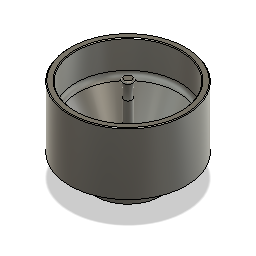
P100_Hot_Load_Funnel (Autodesk Fusion 360 design; units mm, degrees)
Autodesk Fusion 360 part; units mm, degrees
sketch "Sketch1" plane through (0, 0, 0) normal (0, 0, 1) x (1, 0, 0)
  line L0 (0, 0) -> (-35, 0)
  line L1 (-35, 0) -> (-35, 2.5)
  line L2 (-35, 2.5) -> (-39, 2.5)
  line L3 (-39, 2.5) -> (-39, 7.5)
  line L4 (-39, 7.5) -> (-39, 12.5)
  line L5 (-39, 12.5) -> (0, 12.5)
  line L6 (0, 12.5) -> (0, 0)
  line L7 (-39, 12.5) -> (-35, 12.5)
  line L8 (-35, 12.5) -> (-27.7831, 0)
  line L9 (-35.5774, 12.5) -> (-28.3605, 0)
  line L10 (-35, 0) -> (-34, 0) construction
  line L11 (-35, 12.5) -> (-19.3037, -14.6868)
  line L12 (-35.5774, 12.5) -> (-19.8811, -14.6868)
  line L13 (-19.3037, -14.6868) -> (-19.8811, -14.6868)
  line L14 (0, 12.5) -> (-4, 12.5)
  circle A0 centre (-18.149, -12.6868) radius 2
  arc A1 (-18.8484, -10.8131) -> (-4, 20.5) centre (-27.5463, 12.4884) ccw
  line L15 (-19.3037, -14.6868) -> (0, -14.6868)
  line L16 (0, -14.6868) -> (0, 0)
  line L17 (-4, 12.5) -> (-4, 20.5)
  line L18 (0, 12.5) -> (0, 20.5)
  line L19 (0, 20.5) -> (-4, 20.5)
  line L20 (0, 16.5) -> (-3, 16.5)
  line L21 (-39, 12.5) -> (-39, 25.5)
  line L22 (-39, 25.5) -> (0, 25.5)
  line L23 (0, 25.5) -> (0, 20.5)
  line L24 (-4, 20.5) -> (-33, 20.5)
  line L25 (-35, 0) -> (-28.8618, -14.6868)
  line L26 (-28.8618, -14.6868) -> (-19.8811, -14.6868)
  line L27 (-35, 12.5) -> (-35, 19)
  line L28 (-35, 19) -> (-39, 19)
  line L29 (-33, 20.5) -> (-33, 12.5)
  line L30 (-35, 19) -> (0, 19)
  line L31 (-35, 19) -> (-34.8, 19)
  line L32 (-34.8, 19) -> (-34.8, 12.5)
  line L33 (-19.8811, -13.6868) -> (-19.8811, -14.6868)
  line L34 (-18.149, -12.6868) -> (-20.4584, -12.6868)
  line L35 (-28.8618, -14.6868) -> (-28.8618, -26.1449)
  arc A2 (-18.56, -18.617) -> (-19.8811, -13.6868) centre (-28.4205, -18.617) ccw
  line L36 (-18.56, -18.617) -> (-18.56, -22.5613)
  line L37 (-18.56, -22.5613) -> (-28.8618, -22.5613)
  line L38 (-28.8618, -22.5613) -> (-28.8618, -26.1449)
  line L39 (-18.56, -22.5613) -> (0, -22.5613)
  line L40 (0, -22.5613) -> (0, -14.6868)
  line L41 (-19.3771, -14.6868) -> (-28.8618, -14.6868)
  line L42 (-18.56, -22.5613) -> (-21.5, -22.5613)
  line L43 (-21.5, -22.5613) -> (-21.5, -22.1613)
  arc A3 (-21.5, -22.1613) -> (-28.8618, -14.6868) centre (-28.9754, -22.1613) ccw
  circle A4 centre (-18.149, -12.6868) radius 1.8
  line L44 (-20.0811, -12.9897) -> (-20.0811, -14.6868)
  arc A5 (-18.36, -18.617) -> (-20.0811, -12.9897) centre (-28.4205, -18.617) ccw
  line L45 (-18.36, -18.617) -> (-18.36, -22.5613)
  arc A6 (-18.7785, -11.0004) -> (-3.8107, 20.5644) centre (-27.5463, 12.4884) ccw
  line L46 (-39, 7.5) -> (-35, 7.5)
  line L47 (-35, 7.5) -> (-35, 2.5)
  line L48 (-35, 5) -> (-39, 5)
  line L49 (-28.8618, -14.6868) -> (-39, -7.5351)
  line L50 (-35, 0) -> (-35, -10.3567)
  line L51 (-39, 2.5) -> (-39, -7.5351)
  line L52 (-28.8618, -14.6868) -> (-17.6989, -22.5613)
  line L53 (-21.5, -22.5613) -> (-21.5, -19.8799)
  dimension "d1" = 35
  dimension "d4" = 2.5
  dimension "d5" = 4
  dimension "d6" = 5
  dimension "d7" = 5
  dimension "d8" = 4
  dimension "d9" = 120
  dimension "d10" = 0.5
  dimension "d17" = 4
  dimension "d20" = 8
  dimension "d21" = 4
  dimension "d22" = 3
  dimension "d23" = 13
  dimension "d42" = 6.5
  dimension "d43" = 2
  dimension "d44" = 0.2
  dimension "d147" = 4
  dimension "d148" = 2.94
  dimension "d150" = 0.4
  dimension "d151" = -0.2
  dimension "d152" = 0.2
  dimension "d153" = 0.2
  dimension "d168" = 35.2
  dimension "d176" = 21.5
  constraint coincident L0.start L6.end
  constraint horizontal L0
  constraint perpendicular L0 L1
  constraint perpendicular L1 L2
  constraint perpendicular L2 L3
  constraint parallel L3 L4
  constraint perpendicular L4 L5
  constraint perpendicular L5 L6
  constraint perpendicular L4 L7
  constraint coincident L0 L8.end
  constraint coincident L7 L9.start
  constraint coincident L0 L9.end
  constraint parallel L8 L9
  constraint horizontal L10
  constraint parallel L8 L11
  constraint parallel L9 L12
  constraint coincident L12 L13.end
  constraint horizontal L13
  constraint coincident L12.end L13.end
  constraint perpendicular L6 L14
  constraint tangent L11 A0
  constraint perpendicular L0 L16
  constraint perpendicular L14 L17
  constraint perpendicular L14 L18
  constraint coincident L18 L19.start
  constraint horizontal L19
  constraint midpoint L18 L20.start
  constraint coincident A1 L20.end
  constraint perpendicular L18 L20
  constraint perpendicular L7 L21
  constraint perpendicular L21 L22
  constraint perpendicular L19 L23
  constraint perpendicular L17 L24
  constraint parallel L13 L26
  constraint coincident A0 A1.start
  constraint tangent A0 A1
  constraint horizontal L15
  constraint perpendicular L7 L27
  constraint midpoint L21 L28.end
  constraint coincident L5 L29.end
  constraint perpendicular L5 L29
  constraint perpendicular L27 L30
  constraint coincident L18 L30.end
  constraint perpendicular L27 L31
  constraint perpendicular L30 L32
  constraint coincident A0 L33.start
  constraint coincident L26 L12.end
  constraint perpendicular L26 L33
  constraint coincident A0.centre L34.start
  constraint coincident L11 L34.end
  constraint horizontal L34
  constraint tangent A0 L15
  constraint perpendicular L26 L35
  constraint tangent L11 A2
  constraint vertical L36
  constraint tangent A2 L36
  constraint perpendicular L36 L37
  constraint vertical L38
  constraint perpendicular L36 L39
  constraint perpendicular L15 L40
  constraint coincident A2 L41.start
  constraint coincident L13 L41.start
  constraint perpendicular L36 L42
  constraint perpendicular L42 L43
  constraint tangent L43 A3
  constraint perpendicular L4 L46
  constraint midpoint L47 L48.start
  constraint midpoint L3 L48.end
  constraint coincident L49 L50.end
  constraint perpendicular L0 L50
  constraint coincident L1 L0.end
  constraint coincident L49 L51.end
  constraint perpendicular L2 L51
  constraint coincident L39 L52.end
  constraint parallel L49 L52
  constraint coincident L52 L53.end
  constraint perpendicular L42 L53
  measures "d1" distance of L0.start L0.end
  measures "d4" distance of L0.end L1.end
  measures "d5" distance of L1.end L2.end
  measures "d6" distance of L2.end L3.end
  measures "d7" distance of L3.end L4.end
  measures "d8" distance of L4.end L7.end
  measures "d9" angle of L5 L8
  measures "d10" distance of L8 L9
  measures "d17" diameter of A0
  measures "d20" distance of L14.end A1.end
  measures "d21" distance of A1.end L18.end
  measures "d22" distance of L20.start L20.end
  measures "d23" distance of L4.end L21.end
  measures "d42" distance of L7.end L27.end
  measures "d43" distance of L27 L29
  measures "d44" distance of L27.end L31.end
  measures "d147" distance of L11.end A2.start
  measures "d148" distance of L36.end L42.end
  measures "d150" distance of L42.end L43.end
  measures "d168" angle of L15 L49
  measures "d176" distance of L39.end L42.end
revolve "Revolve1" add sketch "Sketch1" angle 360 about axis through (0, 12.5, 0) along (0, -1, 0) contours L0 L11 L12 L44 | L0 L5 L7 L8 L9 L11 L12 | L0 L12 L25 L26 L41 L44 | L0 L1 L4 L5 L7 L9 L12 L46 L47 | L5 L7 L21 L27 L28 | L1 L2 L49 L50 L51 | L25 L49 L50 | L11 L12 L33 L44 | L12 L26 L41 L44 | L2 L3 L47 L48 | L13 L26 A2 L36 L41 A3 L52 | A3 L52 | L13 L33 A2 L41 | L3 L46 L47 L48 | L36 L37 L42 L43 L52 L53 makes body 1
revolve "Revolve2" add sketch "Sketch1" angle 360 about axis through (0, -14.6868, 0) along (0, 1, 0) separate body contours L0 L5 L6 L14 A6 | L0 A0 L15 L16 A6 | A0 A4 A5 A6 | L5 L14 L18 L20 A6 | A4 | L15 L39 L40 A5 L45 L52 | L18 L20 L30 A6 | A0 L15 A5 | L18 L19 L30 A6 | L39 L45 L52 makes body 2
revolve "Revolve3" add sketch "Sketch1" angle 360 about axis through (0, 12.5, 0) along (0, 1, 0) separate body contours L19 L21 L22 L23 L24 L28 L29 L30 L31 | L17 L24 L29 L30 makes body 3
fillet "Fillet1" radius 1 1 edges at (-3.5324, 20.5, 1.3701) on bodies 2
sketch "Sketch2" plane through (0, 19, 0) normal (0, -1, 0) x (1, 0, 0)
  circle A0 centre (0, 0) radius 39
  line L0 (0, 0) -> (39, 0)
  line L1 (39, 0) -> (39, -20)
  circle A1 centre (0, 0) radius 4
  constraint coincident A0.centre L0.start
  constraint coincident A0 L0.end
  constraint horizontal L0
  constraint tangent A0 L1
move_body "Move1" bodies 3 to x (-1, 0, 0) y (0, -1, 0) z (0, 0, 1) at (78, 38, 0)
move_body "Move2" bodies 3 to x (1, 0, 0) y (0, 1, 0) z (0, 0, 1) at (9, 0, 0)
sketch "Sketch4" plane through (0, 19, 0) normal (0, 1, 0) x (-1, 0, 0)
  circle A0 centre (-87, 0) radius 4
  circle A1 centre (-87, 0) radius 39
  line L0 (-87, 0) -> (-48, 0)
  line L1 (-39, 0) -> (-48, 0)
  line L2 (-37.108, 12) -> (-49.892, 12)
  line L3 (-49.892, 12) -> (-49.892, -12)
  line L4 (-49.892, -12) -> (-37.108, -12)
  line L5 (-37.108, -12) -> (-37.108, 12)
  line L6 (-37.108, 12) -> (-49.892, -12) construction
  line L7 (-49.892, 12) -> (-37.108, -12) construction
  circle A2 centre (0, 0) radius 39
  point P0 (-43.5, 0)
  dimension "d70" = 24
  constraint coincident A0.centre A1.centre
  constraint coincident A1 L0.end
  constraint horizontal L0
  constraint parallel L0 L1
  constraint horizontal L2
  constraint perpendicular L2 L3
  constraint parallel L2 L4
  constraint parallel L3 L5
  constraint coincident L6 P0
  constraint coincident L7 P0
  constraint midpoint L1 P0
  constraint coincident L2.start A2
  constraint coincident A1 L2.end
  measures "d70" distance of L2.start L4.end
sketch "Sketch11" plane through (0, 0, -12) normal (0, 0, -1) x (-1, 0, 0)
  line L0 (-47.75, 19) -> (-49.892, 19)
  line L1 (-49.892, 19) -> (-49.892, 12.5)
  line L2 (-49.892, 12.5) -> (-45.7602, 12.5)
  line L3 (-45.7602, 12.5) -> (-45.0052, 13.2448)
  line L4 (-45.0052, 13.2448) -> (-43.5, 14.75)
  arc A0 (-43.5, 14.75) -> (-47.75, 19) centre (-43.5, 19) ccw
  circle A1 centre (-43.5, 19) radius 0.89
  arc A2 (-49.892, 19) -> (-47.75, 19) centre (-48.821, 20.6891) ccw
  dimension "d131" = 2
  constraint coincident L0.start A0.end
  constraint coincident L0.end L1.start
  measures "d131" radius of A2
extrude "Extrude31" cut sketch "Sketch11" against normal blind 40 contours L0 A2 bodies 1 3
sketch "Sketch12" plane through (0, 0, -5.8) normal (0, 0, -1) x (-1, 0, 0)
  circle A0 centre (-43.5, 19) radius 0.89
  arc A1 (-40.6742, 22.1745) -> (-43.5, 14.75) centre (-43.5, 19) ccw
  line L0 (-43.5, 14.75) -> (-41.9948, 13.2242)
  line L1 (-41.9948, 13.2242) -> (-41.9948, 11.4844)
  line L2 (-41.9948, 11.4844) -> (-38.5663, 8.0559)
  line L3 (-38.5663, 8.0559) -> (-38.5663, 19)
  line L4 (-38.5663, 19) -> (-37.108, 19)
  arc A2 (-37.108, 19) -> (-38.5663, 19) centre (-37.8371, 19.6843) ccw
  line L5 (-37.108, 19) -> (-40.6742, 22.1745)
  dimension "d134" = 1
  constraint coincident L3.end L4.start
  constraint coincident L4.end A2.start
  measures "d134" radius of A2
extrude "Extrude32" cut sketch "Sketch12" against normal blind 29 contours L4 A2 L5 | A2 L5 bodies 3 1
sketch "Sketch6" plane through (0, 12.5, 0) normal (0, -1, 0) x (1, 0, 0)
  line L0 (49.892, -12) -> (38.8775, -12)
  line L1 (38.8775, -12) -> (38.8775, -6)
  line L2 (38.8775, -6) -> (49.892, -6)
  line L3 (49.892, -6) -> (49.892, -12)
  line L4 (49.892, 12) -> (38.6774, 12)
  line L5 (38.6774, 12) -> (38.6774, 6)
  line L6 (38.6774, 6) -> (49.892, 6)
  line L7 (49.892, 6) -> (49.892, 12)
  line L8 (49.892, -6.25) -> (38.8775, -6.25)
  line L9 (38.8775, -6.25) -> (38.8775, -5.75)
  line L10 (38.8775, -5.75) -> (49.892, -5.75)
  line L11 (49.892, -5.75) -> (49.892, -6.25)
  line L12 (49.892, -6.25) -> (38.8775, -5.75) construction
  line L13 (38.8775, -6.25) -> (49.892, -5.75) construction
  line L14 (49.892, 6.25) -> (38.6774, 6.25)
  line L15 (38.6774, 6.25) -> (38.6774, 5.75)
  line L16 (38.6774, 5.75) -> (49.892, 5.75)
  line L17 (49.892, 5.75) -> (49.892, 6.25)
  line L18 (49.892, 6.25) -> (38.6774, 5.75) construction
  line L19 (38.6774, 6.25) -> (49.892, 5.75) construction
  circle A0 centre (87, 0) radius 39
  point P0 (44.3848, -6)
  point P1 (44.2847, 6)
  dimension "d75" = 6
  dimension "d76" = 0.5
  dimension "d77" = 0.5
  dimension "d80" = 6
  constraint horizontal L0
  constraint vertical L1
  constraint horizontal L2
  constraint vertical L3
  constraint horizontal L4
  constraint vertical L5
  constraint horizontal L6
  constraint vertical L7
  constraint horizontal L8
  constraint perpendicular L8 L9
  constraint parallel L8 L10
  constraint parallel L9 L11
  constraint coincident L12 P0
  constraint coincident L13 P0
  constraint midpoint L2 P0
  constraint horizontal L14
  constraint perpendicular L14 L15
  constraint parallel L14 L16
  constraint parallel L15 L17
  constraint coincident L18 P1
  constraint coincident L19 P1
  constraint midpoint L6 P1
  measures "d75" distance of L0.start L2.end
  measures "d76" distance of L8.end L9.end
  measures "d77" distance of L14.end L15.end
  measures "d80" distance of L4.start L6.end
sketch "Sketch8" plane through (0, 0, 12) normal (0, 0, 1) x (1, 0, 0)
  line L0 (45.7602, 12.5) -> (49.892, 12.5)
  line L1 (49.892, 12.5) -> (49.892, 19)
  line L2 (43.5, 14.5) -> (48.9179, 19.9656)
  circle A0 centre (43.5, 19) radius 4.5
  arc A1 (47.75, 19) -> (49.892, 19) centre (48.821, 20.6891) ccw
  arc A2 (47.75, 19) -> (43.5, 14.75) centre (43.5, 19) ccw
  line L3 (43.5, 14.75) -> (45.0052, 13.2448)
  line L4 (45.0052, 13.2448) -> (45.7602, 12.5)
  circle A3 centre (43.5, 19) radius 0.89
chamfer "Chamfer5" distance 1 angle 45 1 edges at (48, 12.5, 0) on bodies 3
revolve "Revolve4" add sketch "Sketch1" angle 360 about axis through (0, 12.5, 0) along (0, -1, 0) separate body contours L0 L5 L8 L11 L14 A1 | L0 L11 A0 A1 L34 | L5 L27 L30 L31 L32 | L11 A0 L34 L44 | L5 L14 A1 L17 L30 | L5 L29 L30 L32 | L11 A0 L44 | L5 L17 L29 L30 makes body 4
chamfer "Chamfer8" distance 0.5 angle 45 2 edges at (-32.6315, 19, 12.6565) (-36.3608, 19, 14.103) on bodies 1
sketch "Sketch13" plane through (0, 0, 5.8) normal (0, 0, 1) x (1, 0, 0)
  circle A0 centre (43.5, 19) radius 0.89
  arc A1 (38.5663, 19) -> (38.6013, 20.3293) centre (37.8371, 19.6843) ccw
  line L0 (38.5663, 19) -> (38.0606, 19)
  spline S0 degree 2 poles (38.0606, 19) (38.3118, 18.7516) (38.5663, 18.5) knots 0.145056 0.145056 0.145056 0.216152 0.216152 0.216152 weights 1.000257 1.000277 1.000254
  line L1 (38.5663, 18.5) -> (38.5663, 8.0559)
  line L2 (38.5663, 8.0559) -> (41.9948, 11.4844)
  line L3 (41.9948, 11.4844) -> (41.9948, 13.2242)
  line L4 (41.9948, 13.2242) -> (43.5, 14.75)
  arc A2 (43.5, 14.75) -> (40.6742, 22.1745) centre (43.5, 19) ccw
  line L5 (41.9948, 13.2242) -> (38.5663, 9.7489)
  line L6 (40.6742, 22.1745) -> (38.6013, 20.3293)
  constraint coincident L3.end L4.start
  constraint parallel L4 L5
extrude "Extrude33" cut sketch "Sketch13" against normal blind 20.5 contours L1 L2 L3 L5 bodies 1 3
delete_face "DeleteFace10" 1 faces at (38.5663, 8.6202, -1.9333) on bodies 1
ref_plane "WorkPlane1" through (0, 9, 0) normal (0, 1, 0) x (0, 0, 1)
ref_plane "WorkPlane2" through (0, 12.5, 0) normal (0, 1, 0) x (0, 0, 1)
split "Split3" by plane through (0, 12.5, 0) normal (0, 1, 0) bodies 1 makes body 5 at (-38.8062, 14.5, -3.8831)
split "Split4" by plane through (0, 9, 0) normal (0, 1, 0) bodies 2 makes body 6 at (-1.52, 18.1193, -2.7188)
move_body "Move3" bodies 3 2 to x (1, 0, 0) y (0, 1, 0) z (0, 0, 1) at (0, -15, 0)
move_body "Move4" bodies 1 to x (1, 0, 0) y (0, 1, 0) z (0, 0, 1) at (0, -15, 0)
extrude "Extrude34" add 1 faces at (-37.3912, -2.5, -3.6764) along direction (0, 1, 0) blind 15 on bodies 1 bodies 1 5
extrude "Extrude35" add 1 faces at (1.3451, -6, 0.7977) along direction (0, 1, 0) up to surface (15 mm away) on bodies 2 bodies 2 6
fillet "Fillet11" radius 10 1 edges at (-32.6315, -2.5, 12.6565) on bodies 1
hidden bodies 3 4
equation "d42 = d23 / 2"
named bodies: "Cone", "Stopper", "Lid", "Empty Volume", "Stopper (1)", "Cone (1)"
